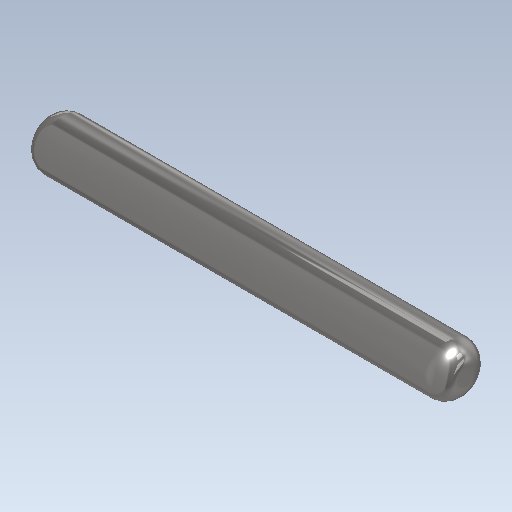
# Autodesk Inventor part: pHHKS25
Saved by Autodesk Inventor 2021 (Build 250183000, 183)
## iProperties
Part Number: pHHKS25
Material: ステンレス鋼
Catalog Web Link: www.cadenas.de
Description: HHKS-pin-Hinges
Vendor: MISUMI
Document SubType Name: Modeling
Designer: partserver
Manufacturer: MISUMI
Mass: 1.38617 g
Surface Area: 2.40777 cm^2
Volume: 0.173272 cm^3
Density: 8 g/cm^3
Appearance: 半つや出し
Category: PARTsolutions
Company: MISUMI
PSOL_IDENT_0: {$CADENAS_DATA\23d-libs\misumi\metric\43_levers_knobs\parts_hhks\hhks_pin.prj},149 {VTYP=3D},{NB=pHH
PSOL_IDENT_1: KS25},{LINA=pHHKS25},{NN=HHKS-pin},{DATE=30.03.2018 07:16:18},{GEOMDATE=17.02.2014},{VERSION=},{LINE
PSOL_IDENT_2: ID=10},{WBVAR=L},{WBNUMERIC=L}  {NB=pHHKS25},{LINA=pHHKS25},{KT=DUMMY},{PN=HHKS25},{MAT=304 Stainles
PSOL_IDENT_3: s Steel},{L=25},{LL=6.0},{L1=13},{L2=0},{L3=0},{NOD=3},{AL=29.4},{WEIGHT=13}
NB: pHHKS25
NN: HHKS-pin
NT: Hinges
NBSYN: p$PN.
LINA: pHHKS25
CATALOG: Misumi
MAT: 304 Stainless Steel
L: 25
SUPPLIER: MISUMI
ARTICLENO: pHHKS25
BOMINFO: pHHKS25
CREATOR: CADENAS GmbH
Title: pHHKS25
Author: Cadenas PARTsolutions
Comments: Hinges
Autodesk Inventor part; units mm, degrees
sketch "Sketch_1" plane through (0, 0, 0) normal (0, 0, 1) x (1, 0, 0)
  line L0 (25, 0) -> (0, 0)
  line L1 (0, 0) -> (0, 0.5)
  arc A0 (1, 1.5) -> (0, 0.5) centre (1, 0.5) ccw
  line L2 (1, 1.5) -> (24, 1.5)
  arc A1 (25, 0.5) -> (24, 1.5) centre (24, 0.5) ccw
  line L3 (25, 0.5) -> (25, 0)
  line L4 (25, 0) -> (0, 0)
  constraints: 10 end point, 4 point on circle, 2 centre point
revolve "Revolution1" add sketch "Sketch_1" angle 360 about axis through (25, 0, 0) along (1, 0, 0)
ref_plane "pin_XY" through (0, 0, 0) normal (1, 0, 0) x (0, 0, -1)
ref_plane "pin_YZ" through (0, 0, 0) normal (0, 0, -1) x (0, 1, 0)
ref_plane "pin_ZX" through (0, 0, 0) normal (0, 1, 0) x (1, 0, 0)
body "Solid1"
